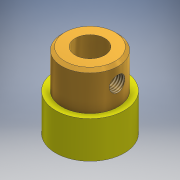
# Autodesk Inventor part: engranePeq
Saved by Autodesk Inventor 2016 (Build 200138000, 138)
## iProperties
Created: 2016-09-20
Part Number: engranePeq
Material: Plástico ABS
Document SubType Name: Modeling
Designer: i95sa
Density: 1.06 g/cm^3
Appearance: Suave - Blanco
Author: i95sa
Autodesk Inventor part; units mm, degrees
ref_plane "YZ Plane" through (0, 0, 0) normal (1, 0, 0) x (0, 1, 0)
ref_plane "XZ Plane" through (0, 0, 0) normal (0, 1, 0) x (-1, 0, 0)
ref_plane "XY Plane" through (0, 0, 0) normal (0, 0, 1) x (1, 0, 0)
sketch "Boceto1" plane through (0, 0, 0) normal (0, 0, 1) x (1, 0, 0)
  circle A0 centre (0, 0) radius 4.75
  circle A1 centre (0, 0) radius 2.5
  dimension "d0" = 9.5
  dimension "d1" = 5
  constraints: 2 centre point, 2 coincident
  measures "d0" diameter of A0
  measures "d1" diameter of A1
extrude "Extrusión1" add sketch "Boceto1" along normal blind 12.7
chamfer "Chaflán1" distance 1 angle 45 1 edges at (-4.75, 0, 0)
chamfer "Chaflán2" distance 0.5 angle 45 1 edges at (-4.75, 0, 12.7)
sketch "Boceto2" plane through (0, 0, 0) normal (0, 0, -1) x (-1, 0, 0)
  circle A0 centre (0, 0) radius 4.75
  arc A1 (-0.1187, -6.799) -> (0.1187, -6.799) centre (0, 0) ccw
  circle A2 centre (0, 0) radius 5.81
  line L0 (0, 0) -> (6, 0) construction
  line L1 (0, 0) -> (6, 0) construction
  line L2 (0, 0) -> (6.8, 0) construction
  line L3 (-0.1187, -6.799) -> (-0.314, -5.9918)
  line L4 (0.314, -5.9918) -> (0.1187, -6.799)
  circle A3 centre (0, 0) radius 4.75 projected
  line L5 (0, 0) -> (6, 0) construction
  circle A4 centre (0, 0) radius 4.25 projected
  line L6 (0, 0) -> (6, 0) construction
  arc A5 (0.314, -5.9918) -> (0.4185, -5.9854) centre (0, 0) ccw
  arc A6 (-0.4185, -5.9854) -> (-0.314, -5.9918) centre (0, 0) ccw
  line L7 (0, 0) -> (6, 0) construction
  arc A7 (0.4185, -5.9854) -> (0.5229, -5.9772) centre (0, 0) ccw
  arc A8 (1.1449, -5.8898) -> (1.2475, -5.8689) centre (0, 0) ccw
  line L8 (1.1449, -5.8898) -> (1.0638, -6.7163)
  arc A9 (0.8287, -6.7493) -> (1.0638, -6.7163) centre (0, 0) ccw
  line L9 (0.8287, -6.7493) -> (0.5229, -5.9772)
  arc A10 (1.2475, -5.8689) -> (1.3497, -5.8462) centre (0, 0) ccw
  arc A11 (1.9534, -5.6731) -> (2.0521, -5.6382) centre (0, 0) ccw
  line L10 (1.9534, -5.6731) -> (1.9881, -6.5029)
  arc A12 (1.76, -6.5683) -> (1.9881, -6.5029) centre (0, 0) ccw
  line L11 (1.76, -6.5683) -> (1.3497, -5.8462)
  arc A13 (2.0521, -5.6382) -> (2.1502, -5.6015) centre (0, 0) ccw
  arc A14 (2.7239, -5.346) -> (2.8168, -5.2977) centre (0, 0) ccw
  line L12 (2.7239, -5.346) -> (2.8738, -6.1629)
  arc A15 (2.657, -6.2594) -> (2.8738, -6.1629) centre (0, 0) ccw
  line L13 (2.657, -6.2594) -> (2.1502, -5.6015)
  arc A16 (2.8168, -5.2977) -> (2.9089, -5.2477) centre (0, 0) ccw
  arc A17 (3.4415, -4.9149) -> (3.5267, -4.8541) centre (0, 0) ccw
  line L14 (3.4415, -4.9149) -> (3.7035, -5.703)
  arc A18 (3.5023, -5.8287) -> (3.7035, -5.703) centre (0, 0) ccw
  line L15 (3.5023, -5.8287) -> (2.9089, -5.2477)
  arc A19 (3.5267, -4.8541) -> (3.6109, -4.7918) centre (0, 0) ccw
  arc A20 (4.092, -4.3881) -> (4.168, -4.316) centre (0, 0) ccw
  line L16 (4.092, -4.3881) -> (4.4612, -5.132)
  arc A21 (4.2794, -5.2846) -> (4.4612, -5.132) centre (0, 0) ccw
  line L17 (4.2794, -5.2846) -> (3.6109, -4.7918)
  arc A22 (4.168, -4.316) -> (4.2426, -4.2426) centre (0, 0) ccw
  arc A23 (4.6629, -3.7759) -> (4.7281, -3.694) centre (0, 0) ccw
  line L18 (4.6629, -3.7759) -> (5.132, -4.4612)
  arc A24 (4.9732, -4.6376) -> (5.132, -4.4612) centre (0, 0) ccw
  line L19 (4.9732, -4.6376) -> (4.2426, -4.2426)
  arc A25 (4.7281, -3.694) -> (4.7918, -3.6109) centre (0, 0) ccw
  arc A26 (5.143, -3.0902) -> (5.1962, -3) centre (0, 0) ccw
  line L20 (5.143, -3.0902) -> (5.703, -3.7035)
  arc A27 (5.5702, -3.9003) -> (5.703, -3.7035) centre (0, 0) ccw
  line L21 (5.5702, -3.9003) -> (4.7918, -3.6109)
  arc A28 (5.1962, -3) -> (5.2477, -2.9089) centre (0, 0) ccw
  arc A29 (5.523, -2.3444) -> (5.5631, -2.2476) centre (0, 0) ccw
  line L22 (5.523, -2.3444) -> (6.1629, -2.8738)
  arc A30 (6.0588, -3.0871) -> (6.1629, -2.8738) centre (0, 0) ccw
  line L23 (6.0588, -3.0871) -> (5.2477, -2.9089)
  arc A31 (5.5631, -2.2476) -> (5.6015, -2.1502) centre (0, 0) ccw
  arc A32 (5.7956, -1.5529) -> (5.8218, -1.4515) centre (0, 0) ccw
  line L24 (5.7956, -1.5529) -> (6.5029, -1.9881)
  arc A33 (6.4295, -2.2139) -> (6.5029, -1.9881) centre (0, 0) ccw
  line L25 (6.4295, -2.2139) -> (5.6015, -2.1502)
  arc A34 (5.8218, -1.4515) -> (5.8462, -1.3497) centre (0, 0) ccw
  arc A35 (5.9553, -0.7312) -> (5.9671, -0.6272) centre (0, 0) ccw
  line L26 (5.9553, -0.7312) -> (6.7163, -1.0638)
  arc A36 (6.6751, -1.2975) -> (6.7163, -1.0638) centre (0, 0) ccw
  line L27 (6.6751, -1.2975) -> (5.8462, -1.3497)
  arc A37 (5.9671, -0.6272) -> (5.9772, -0.5229) centre (0, 0) ccw
  arc A38 (5.9991, 0.1047) -> (5.9963, 0.2094) centre (0, 0) ccw
  line L28 (5.9991, 0.1047) -> (6.799, -0.1187)
  arc A39 (6.7907, -0.3559) -> (6.799, -0.1187) centre (0, 0) ccw
  line L29 (6.7907, -0.3559) -> (5.9772, -0.5229)
  arc A40 (5.9963, 0.2094) -> (5.9918, 0.314) centre (0, 0) ccw
  arc A41 (5.9261, 0.9386) -> (5.9088, 1.0419) centre (0, 0) ccw
  line L30 (5.9261, 0.9386) -> (6.7493, 0.8287)
  arc A42 (6.7741, 0.5927) -> (6.7493, 0.8287) centre (0, 0) ccw
  line L31 (6.7741, 0.5927) -> (5.9918, 0.314)
  arc A43 (5.9088, 1.0419) -> (5.8898, 1.1449) centre (0, 0) ccw
  arc A44 (5.7378, 1.7542) -> (5.7063, 1.8541) centre (0, 0) ccw
  line L32 (5.7378, 1.7542) -> (6.5683, 1.76)
  arc A45 (6.6257, 1.5297) -> (6.5683, 1.76) centre (0, 0) ccw
  line L33 (6.6257, 1.5297) -> (5.8898, 1.1449)
  arc A46 (5.7063, 1.8541) -> (5.6731, 1.9534) centre (0, 0) ccw
  arc A47 (5.4378, 2.5357) -> (5.3928, 2.6302) centre (0, 0) ccw
  line L34 (5.4378, 2.5357) -> (6.2594, 2.657)
  arc A48 (6.3483, 2.4369) -> (6.2594, 2.657) centre (0, 0) ccw
  line L35 (6.3483, 2.4369) -> (5.6731, 1.9534)
  arc A49 (5.3928, 2.6302) -> (5.346, 2.7239) centre (0, 0) ccw
  arc A50 (5.032, 3.2678) -> (4.9742, 3.3552) centre (0, 0) ccw
  line L36 (5.032, 3.2678) -> (5.8287, 3.5023)
  arc A51 (5.9474, 3.2967) -> (5.8287, 3.5023) centre (0, 0) ccw
  line L37 (5.9474, 3.2967) -> (5.346, 2.7239)
  arc A52 (4.9742, 3.3552) -> (4.9149, 3.4415) centre (0, 0) ccw
  arc A53 (4.5283, 3.9364) -> (4.4589, 4.0148) centre (0, 0) ccw
  line L38 (4.5283, 3.9364) -> (5.2846, 4.2794)
  arc A54 (5.4307, 4.0923) -> (5.2846, 4.2794) centre (0, 0) ccw
  line L39 (5.4307, 4.0923) -> (4.9149, 3.4415)
  arc A55 (4.4589, 4.0148) -> (4.3881, 4.092) centre (0, 0) ccw
  arc A56 (3.9364, 4.5283) -> (3.8567, 4.5963) centre (0, 0) ccw
  line L40 (3.9364, 4.5283) -> (4.6376, 4.9732)
  arc A57 (4.8083, 4.8083) -> (4.6376, 4.9732) centre (0, 0) ccw
  line L41 (4.8083, 4.8083) -> (4.3881, 4.092)
  arc A58 (3.8567, 4.5963) -> (3.7759, 4.6629) centre (0, 0) ccw
  arc A59 (3.2678, 5.032) -> (3.1795, 5.0883) centre (0, 0) ccw
  line L42 (3.2678, 5.032) -> (3.9003, 5.5702)
  arc A60 (4.0923, 5.4307) -> (3.9003, 5.5702) centre (0, 0) ccw
  line L43 (4.0923, 5.4307) -> (3.7759, 4.6629)
  arc A61 (3.1795, 5.0883) -> (3.0902, 5.143) centre (0, 0) ccw
  arc A62 (2.5357, 5.4378) -> (2.4404, 5.4813) centre (0, 0) ccw
  line L44 (2.5357, 5.4378) -> (3.0871, 6.0588)
  arc A63 (3.2967, 5.9474) -> (3.0871, 6.0588) centre (0, 0) ccw
  line L45 (3.2967, 5.9474) -> (3.0902, 5.143)
  arc A64 (2.4404, 5.4813) -> (2.3444, 5.523) centre (0, 0) ccw
  arc A65 (1.7542, 5.7378) -> (1.6538, 5.7676) centre (0, 0) ccw
  line L46 (1.7542, 5.7378) -> (2.2139, 6.4295)
  arc A66 (2.4369, 6.3483) -> (2.2139, 6.4295) centre (0, 0) ccw
  line L47 (2.4369, 6.3483) -> (2.3444, 5.523)
  arc A67 (1.6538, 5.7676) -> (1.5529, 5.7956) centre (0, 0) ccw
  arc A68 (0.9386, 5.9261) -> (0.835, 5.9416) centre (0, 0) ccw
  line L48 (0.9386, 5.9261) -> (1.2975, 6.6751)
  arc A69 (1.5297, 6.6257) -> (1.2975, 6.6751) centre (0, 0) ccw
  line L49 (1.5297, 6.6257) -> (1.5529, 5.7956)
  arc A70 (0.835, 5.9416) -> (0.7312, 5.9553) centre (0, 0) ccw
  arc A71 (0.1047, 5.9991) -> (0, 6) centre (0, 0) ccw
  line L50 (0.1047, 5.9991) -> (0.3559, 6.7907)
  arc A72 (0.5927, 6.7741) -> (0.3559, 6.7907) centre (0, 0) ccw
  line L51 (0.5927, 6.7741) -> (0.7312, 5.9553)
  arc A73 (0, 6) -> (-0.1047, 5.9991) centre (0, 0) ccw
  arc A74 (-0.7312, 5.9553) -> (-0.835, 5.9416) centre (0, 0) ccw
  line L52 (-0.7312, 5.9553) -> (-0.5927, 6.7741)
  arc A75 (-0.3559, 6.7907) -> (-0.5927, 6.7741) centre (0, 0) ccw
  line L53 (-0.3559, 6.7907) -> (-0.1047, 5.9991)
  arc A76 (-0.835, 5.9416) -> (-0.9386, 5.9261) centre (0, 0) ccw
  arc A77 (-1.5529, 5.7956) -> (-1.6538, 5.7676) centre (0, 0) ccw
  line L54 (-1.5529, 5.7956) -> (-1.5297, 6.6257)
  arc A78 (-1.2975, 6.6751) -> (-1.5297, 6.6257) centre (0, 0) ccw
  line L55 (-1.2975, 6.6751) -> (-0.9386, 5.9261)
  arc A79 (-1.6538, 5.7676) -> (-1.7542, 5.7378) centre (0, 0) ccw
  arc A80 (-2.3444, 5.523) -> (-2.4404, 5.4813) centre (0, 0) ccw
  line L56 (-2.3444, 5.523) -> (-2.4369, 6.3483)
  arc A81 (-2.2139, 6.4295) -> (-2.4369, 6.3483) centre (0, 0) ccw
  line L57 (-2.2139, 6.4295) -> (-1.7542, 5.7378)
  arc A82 (-2.4404, 5.4813) -> (-2.5357, 5.4378) centre (0, 0) ccw
  arc A83 (-3.0902, 5.143) -> (-3.1795, 5.0883) centre (0, 0) ccw
  line L58 (-3.0902, 5.143) -> (-3.2967, 5.9474)
  arc A84 (-3.0871, 6.0588) -> (-3.2967, 5.9474) centre (0, 0) ccw
  line L59 (-3.0871, 6.0588) -> (-2.5357, 5.4378)
  arc A85 (-3.1795, 5.0883) -> (-3.2678, 5.032) centre (0, 0) ccw
  arc A86 (-3.7759, 4.6629) -> (-3.8567, 4.5963) centre (0, 0) ccw
  line L60 (-3.7759, 4.6629) -> (-4.0923, 5.4307)
  arc A87 (-3.9003, 5.5702) -> (-4.0923, 5.4307) centre (0, 0) ccw
  line L61 (-3.9003, 5.5702) -> (-3.2678, 5.032)
  arc A88 (-3.8567, 4.5963) -> (-3.9364, 4.5283) centre (0, 0) ccw
  arc A89 (-4.3881, 4.092) -> (-4.4589, 4.0148) centre (0, 0) ccw
  line L62 (-4.3881, 4.092) -> (-4.8083, 4.8083)
  arc A90 (-4.6376, 4.9732) -> (-4.8083, 4.8083) centre (0, 0) ccw
  line L63 (-4.6376, 4.9732) -> (-3.9364, 4.5283)
  arc A91 (-4.4589, 4.0148) -> (-4.5283, 3.9364) centre (0, 0) ccw
  arc A92 (-4.9149, 3.4415) -> (-4.9742, 3.3552) centre (0, 0) ccw
  line L64 (-4.9149, 3.4415) -> (-5.4307, 4.0923)
  arc A93 (-5.2846, 4.2794) -> (-5.4307, 4.0923) centre (0, 0) ccw
  line L65 (-5.2846, 4.2794) -> (-4.5283, 3.9364)
  arc A94 (-4.9742, 3.3552) -> (-5.032, 3.2678) centre (0, 0) ccw
  arc A95 (-5.346, 2.7239) -> (-5.3928, 2.6302) centre (0, 0) ccw
  line L66 (-5.346, 2.7239) -> (-5.9474, 3.2967)
  arc A96 (-5.8287, 3.5023) -> (-5.9474, 3.2967) centre (0, 0) ccw
  line L67 (-5.8287, 3.5023) -> (-5.032, 3.2678)
  arc A97 (-5.3928, 2.6302) -> (-5.4378, 2.5357) centre (0, 0) ccw
  arc A98 (-5.6731, 1.9534) -> (-5.7063, 1.8541) centre (0, 0) ccw
  line L68 (-5.6731, 1.9534) -> (-6.3483, 2.4369)
  arc A99 (-6.2594, 2.657) -> (-6.3483, 2.4369) centre (0, 0) ccw
  line L69 (-6.2594, 2.657) -> (-5.4378, 2.5357)
  arc A100 (-5.7063, 1.8541) -> (-5.7378, 1.7542) centre (0, 0) ccw
  arc A101 (-5.8898, 1.1449) -> (-5.9088, 1.0419) centre (0, 0) ccw
  line L70 (-5.8898, 1.1449) -> (-6.6257, 1.5297)
  arc A102 (-6.5683, 1.76) -> (-6.6257, 1.5297) centre (0, 0) ccw
  line L71 (-6.5683, 1.76) -> (-5.7378, 1.7542)
  arc A103 (-5.9088, 1.0419) -> (-5.9261, 0.9386) centre (0, 0) ccw
  arc A104 (-5.9918, 0.314) -> (-5.9963, 0.2094) centre (0, 0) ccw
  line L72 (-5.9918, 0.314) -> (-6.7741, 0.5927)
  arc A105 (-6.7493, 0.8287) -> (-6.7741, 0.5927) centre (0, 0) ccw
  line L73 (-6.7493, 0.8287) -> (-5.9261, 0.9386)
  arc A106 (-5.9963, 0.2094) -> (-5.9991, 0.1047) centre (0, 0) ccw
  arc A107 (-5.9772, -0.5229) -> (-5.9671, -0.6272) centre (0, 0) ccw
  line L74 (-5.9772, -0.5229) -> (-6.7907, -0.3559)
  arc A108 (-6.799, -0.1187) -> (-6.7907, -0.3559) centre (0, 0) ccw
  line L75 (-6.799, -0.1187) -> (-5.9991, 0.1047)
  arc A109 (-5.9671, -0.6272) -> (-5.9553, -0.7312) centre (0, 0) ccw
  arc A110 (-5.8462, -1.3497) -> (-5.8218, -1.4515) centre (0, 0) ccw
  line L76 (-5.8462, -1.3497) -> (-6.6751, -1.2975)
  arc A111 (-6.7163, -1.0638) -> (-6.6751, -1.2975) centre (0, 0) ccw
  line L77 (-6.7163, -1.0638) -> (-5.9553, -0.7312)
  arc A112 (-5.8218, -1.4515) -> (-5.7956, -1.5529) centre (0, 0) ccw
  arc A113 (-5.6015, -2.1502) -> (-5.5631, -2.2476) centre (0, 0) ccw
  line L78 (-5.6015, -2.1502) -> (-6.4295, -2.2139)
  arc A114 (-6.5029, -1.9881) -> (-6.4295, -2.2139) centre (0, 0) ccw
  line L79 (-6.5029, -1.9881) -> (-5.7956, -1.5529)
  arc A115 (-5.5631, -2.2476) -> (-5.523, -2.3444) centre (0, 0) ccw
  arc A116 (-5.2477, -2.9089) -> (-5.1962, -3) centre (0, 0) ccw
  line L80 (-5.2477, -2.9089) -> (-6.0588, -3.0871)
  arc A117 (-6.1629, -2.8738) -> (-6.0588, -3.0871) centre (0, 0) ccw
  line L81 (-6.1629, -2.8738) -> (-5.523, -2.3444)
  arc A118 (-5.1962, -3) -> (-5.143, -3.0902) centre (0, 0) ccw
  arc A119 (-4.7918, -3.6109) -> (-4.7281, -3.694) centre (0, 0) ccw
  line L82 (-4.7918, -3.6109) -> (-5.5702, -3.9003)
  arc A120 (-5.703, -3.7035) -> (-5.5702, -3.9003) centre (0, 0) ccw
  line L83 (-5.703, -3.7035) -> (-5.143, -3.0902)
  arc A121 (-4.7281, -3.694) -> (-4.6629, -3.7759) centre (0, 0) ccw
  arc A122 (-4.2426, -4.2426) -> (-4.168, -4.316) centre (0, 0) ccw
  line L84 (-4.2426, -4.2426) -> (-4.9732, -4.6376)
  arc A123 (-5.132, -4.4612) -> (-4.9732, -4.6376) centre (0, 0) ccw
  line L85 (-5.132, -4.4612) -> (-4.6629, -3.7759)
  arc A124 (-4.168, -4.316) -> (-4.092, -4.3881) centre (0, 0) ccw
  arc A125 (-3.6109, -4.7918) -> (-3.5267, -4.8541) centre (0, 0) ccw
  line L86 (-3.6109, -4.7918) -> (-4.2794, -5.2846)
  arc A126 (-4.4612, -5.132) -> (-4.2794, -5.2846) centre (0, 0) ccw
  line L87 (-4.4612, -5.132) -> (-4.092, -4.3881)
  arc A127 (-3.5267, -4.8541) -> (-3.4415, -4.9149) centre (0, 0) ccw
  arc A128 (-2.9089, -5.2477) -> (-2.8168, -5.2977) centre (0, 0) ccw
  line L88 (-2.9089, -5.2477) -> (-3.5023, -5.8287)
  arc A129 (-3.7035, -5.703) -> (-3.5023, -5.8287) centre (0, 0) ccw
  line L89 (-3.7035, -5.703) -> (-3.4415, -4.9149)
  arc A130 (-2.8168, -5.2977) -> (-2.7239, -5.346) centre (0, 0) ccw
  arc A131 (-2.1502, -5.6015) -> (-2.0521, -5.6382) centre (0, 0) ccw
  line L90 (-2.1502, -5.6015) -> (-2.657, -6.2594)
  arc A132 (-2.8738, -6.1629) -> (-2.657, -6.2594) centre (0, 0) ccw
  line L91 (-2.8738, -6.1629) -> (-2.7239, -5.346)
  arc A133 (-2.0521, -5.6382) -> (-1.9534, -5.6731) centre (0, 0) ccw
  arc A134 (-1.3497, -5.8462) -> (-1.2475, -5.8689) centre (0, 0) ccw
  line L92 (-1.3497, -5.8462) -> (-1.76, -6.5683)
  arc A135 (-1.9881, -6.5029) -> (-1.76, -6.5683) centre (0, 0) ccw
  line L93 (-1.9881, -6.5029) -> (-1.9534, -5.6731)
  arc A136 (-1.2475, -5.8689) -> (-1.1449, -5.8898) centre (0, 0) ccw
  arc A137 (-0.5229, -5.9772) -> (-0.4185, -5.9854) centre (0, 0) ccw
  line L94 (-0.5229, -5.9772) -> (-0.8287, -6.7493)
  arc A138 (-1.0638, -6.7163) -> (-0.8287, -6.7493) centre (0, 0) ccw
  line L95 (-1.0638, -6.7163) -> (-1.1449, -5.8898)
  dimension "d11" = 11.62
  dimension "d29" = 360
  constraints: 270 point on circle, 192 end point, 137 centre point, 6 horizontal, 4 coincident, 586 other
  measures "d11" diameter of A2
extrude "Extrusión2" add sketch "Boceto2" against normal blind 6.25 contours A2
sketch "Boceto3" plane through (0, 0, 0) normal (1, 0, 0) x (0, 1, 0)
  circle A0 centre (0, 9.6574) radius 1.3059
  point P0 (0, 0)
  constraints: 1 centre point
extrude "Extrusión3" cut sketch "Boceto3" along normal blind 10
thread "Rosca1" size "M2x0.4" class "6H" standard "ANSI Metric M Profile" full length
